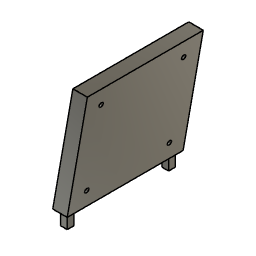
WRO Camera v3 (1) (Autodesk Fusion 360 design; units mm, degrees)
Autodesk Fusion 360 part; units mm, degrees
note: some values were not read from the file. Set by a fixed rule: which sketch regions a step uses.
sketch "Sketch1" plane through (0, 0, 0) normal (0, 1, 0) x (1, 0, 0)
  line L0 (0, 0) -> (6.9459, -39.3923)
  line L1 (0, 0) -> (40, 0) construction
  line L2 (0, 0) -> (5, 0)
  line L3 (6.9459, -39.3923) -> (11.9459, -39.3923)
  line L4 (5, 0) -> (11.9459, -39.3923)
  dimension "d1" = 80
  dimension "d2" = 40
  dimension "d3" = 5
  dimension "d4" = 5
  constraint horizontal L1
  constraint coincident L0.start L1.start
  constraint parallel L1 L2
  constraint horizontal L3
  measures "d1" angle of L0 L1
  measures "d2" distance of L0.start L0.end
  measures "d3" distance of L0.start L2.end
  measures "d4" distance of L0.end L3.end
extrude "Extrude1" add sketch "Sketch1" along normal blind 40
sketch "Sketch2" plane through (0, 0, 0) normal (0, 0, -1) x (1, 0, 0)
  line L0 (5, 0) -> (0, 0)
  line L1 (0, 0) -> (0, -40)
  line L2 (0, -40) -> (5, -40)
  line L3 (5, -40) -> (5, 0)
  line L4 (0, -40) -> (0, -38.75)
  line L5 (0, -38.75) -> (0, -38.65)
  line L6 (0, -38.65) -> (1.35, -38.65)
  line L7 (1.35, -38.65) -> (3.65, -38.65)
  line L8 (3.65, -38.65) -> (3.65, -36.35)
  line L9 (3.65, -36.35) -> (1.35, -36.35)
  line L10 (1.35, -36.35) -> (1.35, -38.65)
  line L11 (0, 0) -> (0, -1.35)
  line L12 (0, -1.35) -> (1.35, -1.35)
  line L13 (1.35, -1.35) -> (3.65, -1.35)
  line L14 (3.65, -1.35) -> (3.65, -3.65)
  line L15 (3.65, -3.65) -> (1.35, -3.65)
  line L16 (1.35, -3.65) -> (1.35, -1.35)
  dimension "d7" = 1.25
  dimension "d8" = 0.1
  dimension "d9" = 1.35
  dimension "d10" = 2.3
  dimension "d11" = 2.3
  dimension "d12" = 1.35
  dimension "d13" = 1.35
  dimension "d14" = 2.3
  dimension "d15" = 2.3
  constraint coincident L1.end L2.start
  constraint perpendicular L2 L4
  constraint vertical L5
  constraint perpendicular L5 L6
  constraint horizontal L7
  constraint vertical L8
  constraint horizontal L9
  constraint vertical L10
  constraint coincident L0.end L1.start
  constraint perpendicular L0 L11
  constraint perpendicular L11 L12
  constraint horizontal L13
  constraint vertical L14
  constraint horizontal L15
  constraint vertical L16
  measures "d7" distance of L1.end L4.end
  measures "d8" distance of L4.end L5.end
  measures "d9" distance of L5.end L6.end
  measures "d10" distance of L6.end L7.end
  measures "d11" distance of L6.end L9.end
  measures "d12" distance of L0.end L11.end
  measures "d13" distance of L11.end L12.end
  measures "d14" distance of L12.end L13.end
  measures "d15" distance of L12.end L15.end
extrude "Extrude2" add sketch "Sketch2" along normal blind 5 contours L7 L8 L9 L10 | L13 L14 L15 L16
sketch "Sketch3" plane through (4.8492, 0, -0.8551) normal (0.984808, 0, -0.173648) x (0, 1, 0)
  line L0 (0, 40.8682) -> (0, 0.8682)
  line L1 (0, 0.8682) -> (40, 0.8682)
  line L2 (40, 0.8682) -> (40, 40.8682)
  line L3 (40, 40.8682) -> (0, 40.8682)
  line L4 (5.9613, 40.8682) -> (5.9613, 35.8682)
  line L5 (0, 35.8688) -> (5, 35.8688)
  line L6 (5, 35.8688) -> (5, 35.1188)
  line L7 (5, 35.1188) -> (5.75, 35.1188)
  circle A0 centre (5.75, 35.1188) radius 0.75
  line L8 (5.75, 35.1188) -> (34.25, 35.1188)
  circle A1 centre (34.25, 35.1188) radius 0.75
  line L9 (5.75, 35.1188) -> (5.75, 6.6188)
  circle A2 centre (5.75, 6.6188) radius 0.75
  line L10 (5.75, 6.6188) -> (34.25, 6.6188)
  circle A3 centre (34.25, 6.6188) radius 0.75
  dimension "d18" = 5
  dimension "d19" = 5
  dimension "d20" = 0.75
  dimension "d21" = 0.75
  dimension "d22" = 1.5
  dimension "d23" = 28.5
  dimension "d24" = 1.5
  dimension "d25" = 28.5
  dimension "d26" = 1.5
  dimension "d27" = 28.5
  dimension "d28" = 1.5
  constraint coincident L3 L4.start
  constraint perpendicular L3 L4
  constraint coincident L0 L5.start
  constraint perpendicular L0 L5
  constraint perpendicular L5 L6
  constraint perpendicular L6 L7
  constraint coincident L7.end A0.centre
  constraint perpendicular L2 L8
  constraint coincident L8.end A1.centre
  constraint perpendicular L1 L9
  constraint coincident L9.end A2.centre
  constraint perpendicular L9 L10
  constraint coincident L10.end A3.centre
  measures "d18" distance of L4.start L4.end
  measures "d19" distance of L5.start L5.end
  measures "d20" distance of L5.end L6.end
  measures "d21" distance of L6.end L7.end
  measures "d22" diameter of A0
  measures "d23" distance of L7.end L8.end
  measures "d24" diameter of A1
  measures "d25" distance of L7.end L9.end
  measures "d26" diameter of A2
  measures "d27" distance of L9.end L10.end
  measures "d28" diameter of A3
extrude "Extrude3" cut sketch "Sketch3" against normal blind 7098 contours L7 A0 L8 | L7 A0 L9 | A0 L8 L9 | A1 | L9 A2 L10 | L9 A2 L10 | A3
